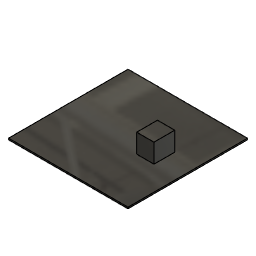
case (Autodesk Fusion 360 archive; units mm, degrees)
design "trill_square"
Autodesk Fusion 360 part; units mm, degrees
sketch "Sketch1" plane through (0, 0, 0) normal (0, 1, 0) x (1, 0, 0)
  line L0 (34.5, -34.5) -> (-34.5, -34.5)
  line L1 (-34.5, -34.5) -> (-34.5, 34.5)
  line L2 (-34.5, 34.5) -> (34.5, 34.5)
  line L3 (34.5, 34.5) -> (34.5, -34.5)
  line L4 (34.5, -34.5) -> (-34.5, 34.5) construction
  line L5 (-34.5, -34.5) -> (34.5, 34.5) construction
  line L6 (15.5, 34.5) -> (15.5, -34.5)
  line L7 (20.5, -6) -> (10.5, -6)
  line L8 (10.5, -6) -> (10.5, 6)
  line L9 (10.5, 6) -> (20.5, 6)
  line L10 (20.5, 6) -> (20.5, -6)
  line L11 (20.5, -6) -> (10.5, 6) construction
  line L12 (10.5, -6) -> (20.5, 6) construction
  line L13 (10.5, 6.5) -> (20.5, 6.5)
  line L14 (20.5, -5.5) -> (10.5, -5.5)
  line L15 (10.5, 6.5) -> (10.5, -5.5)
  line L16 (10.5, -5.5) -> (20.5, -5.5)
  line L17 (20.5, -5.5) -> (20.5, 6.5)
  line L18 (20.5, 6.5) -> (10.5, 6.5)
  point P0 (15.5, 0)
  dimension "d1" = 69
  dimension "d2" = 69
  dimension "d3" = 19
  dimension "d4" = 10
  dimension "d5" = 12
  dimension "d6" = -0.5
  dimension "d7" = 0.5
  constraint horizontal L0
  constraint perpendicular L0 L1
  constraint parallel L0 L2
  constraint parallel L1 L3
  constraint coincident L4 origin
  constraint coincident L5 origin
  constraint coincident L2 L6.start
  constraint coincident L0 L6.end
  constraint perpendicular L0 L6
  constraint horizontal L7
  constraint perpendicular L7 L8
  constraint parallel L7 L9
  constraint parallel L8 L10
  constraint coincident L11 P0
  constraint coincident L12 P0
  constraint midpoint L6 P0
  constraint perpendicular L15 L16
  constraint parallel L15 L17
  constraint parallel L16 L18
  constraint perpendicular L14 L15
  measures "d1" distance of L1.end L2.end
  measures "d2" distance of L0.end L1.end
  measures "d3" distance of L3 L6
  measures "d4" distance of L8.end L9.end
  measures "d5" distance of L7.end L8.end
extrude "Extrude1" add sketch "Sketch1" against normal blind 0.8
extrude "Extrude2" add sketch "Sketch1" along normal blind 11 contours L6 L8 L9 L14 L15 L16 | L6 L9 L10 L14 L16 L17 | L6 L9 L13 L17 L18 | L6 L9 L13 L15 L18

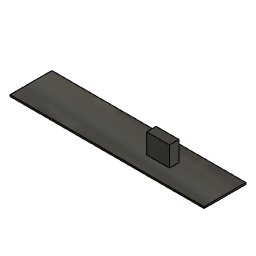
design "trill_bar"
Autodesk Fusion 360 part; units mm, degrees
sketch "Sketch1" plane through (0, 0, 0) normal (0, 1, 0) x (1, 0, 0)
  line L0 (51, -11) -> (-51, -11)
  line L1 (-51, -11) -> (-51, 11)
  line L2 (-51, 11) -> (51, 11)
  line L3 (51, 11) -> (51, -11)
  line L4 (51, -11) -> (-51, 11) construction
  line L5 (-51, -11) -> (51, 11) construction
  line L6 (24.3, 11) -> (24.3, -11)
  line L7 (24.3, 0) -> (12.3, 0)
  line L8 (12.3, 0) -> (12.3, 2.5)
  line L9 (12.3, 2.5) -> (24.3, 2.5)
  line L10 (12.3, 0) -> (12.3, -2.5)
  line L11 (12.3, -2.5) -> (24.3, -2.5)
  dimension "d1" = 102
  dimension "d2" = 22
  dimension "d3" = 26.7
  dimension "d4" = 12
  dimension "d5" = 2.5
  constraint horizontal L0
  constraint perpendicular L0 L1
  constraint parallel L0 L2
  constraint parallel L1 L3
  constraint coincident L4 origin
  constraint coincident L5 origin
  constraint coincident L2 L6.start
  constraint coincident L0 L6.end
  constraint perpendicular L0 L6
  constraint midpoint L6 L7.start
  constraint perpendicular L6 L7
  constraint perpendicular L7 L8
  constraint coincident L6 L9.end
  constraint perpendicular L6 L9
  constraint symmetric L8.start L7 L10.start
  constraint symmetric L7 L8.end L10.end
  constraint symmetric L7 L9.end L11.end
  measures "d1" distance of L1.end L2.end
  measures "d2" distance of L0.end L1.end
  measures "d3" distance of L3 L6
  measures "d4" distance of L7.start L7.end
  measures "d5" distance of L7.end L8.end
extrude "Extrude1" add sketch "Sketch1" against normal blind 0.8
extrude "Extrude2" add sketch "Sketch1" along normal blind 10.5 contours L6 L7 L10 L11 | L6 L7 L8 L9

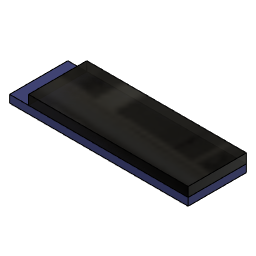
design "oled"
Autodesk Fusion 360 part; units mm, degrees
sketch "Sketch1" plane through (0, 0, 0) normal (0, 1, 0) x (1, 0, 0)
  line L0 (18.85, -6.15) -> (-18.85, -6.15)
  line L1 (-18.85, -6.15) -> (-18.85, 6.15)
  line L2 (-18.85, 6.15) -> (18.85, 6.15)
  line L3 (18.85, 6.15) -> (18.85, -6.15)
  line L4 (18.85, -6.15) -> (-18.85, 6.15) construction
  line L5 (-18.85, -6.15) -> (18.85, 6.15) construction
  dimension "d1" = 37.7
  dimension "d2" = 12.3
  constraint horizontal L0
  constraint perpendicular L0 L1
  constraint parallel L0 L2
  constraint parallel L1 L3
  constraint coincident L4 origin
  constraint coincident L5 origin
  measures "d1" distance of L1.end L2.end
  measures "d2" distance of L0.end L1.end
extrude "Extrude1" add sketch "Sketch1" along normal blind 1.6 makes body 1
sketch "Sketch2" plane through (0, 1.6, 0) normal (0, 1, 0) x (-1, 0, 0)
  line L0 (-18.85, -6.15) -> (18.85, -6.15)
  line L1 (18.85, -6.15) -> (18.85, 6.15)
  line L2 (18.85, 6.15) -> (-18.85, 6.15)
  line L3 (-18.85, 6.15) -> (-18.85, -6.15)
  line L4 (14.85, -6.15) -> (14.85, 6.15)
  dimension "d5" = 4
  constraint coincident L0 L4.start
  constraint coincident L2 L4.end
  constraint perpendicular L2 L4
  measures "d5" distance of L1 L4
extrude "Extrude2" add sketch "Sketch2" along normal blind 2 contours L0 L2 L3 L4 bodies 1
split "Split1" by plane through (0, 1.6, 0) normal (0, 1, 0) bodies 1 makes body 2 at (7.6167, 3.6, 2.05)
equation "d6 = 3.7 mm - 1.7 mm"
